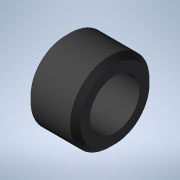
# Autodesk Inventor part: CLBUS5-8-5
Saved by Autodesk Inventor 2021 (Build 250183000, 183)
## iProperties
Created: 2025-06-10
Part Number: CLBUS5-8-5
Material: Generic
Catalog Web Link: www.cadenas.de
Description: CLBU, CLBUB, CLBUM, CLBUS,  CLBP, CLBPB, CLBPM, CLBPS-Bearing Spacers - For Inner Ring
Vendor: MISUMI
Document SubType Name: Modeling
Designer: psAdmin
Manufacturer: MISUMI
Mass: 0.147131 g
Surface Area: 2.50092 cm^2
Volume: 0.147131 cm^3
Density: 1 g/cm^3
Appearance: PSOLRGB-191-191-191
Category: PARTsolutions
Company: MISUMI
Title: CLBUS5-8-5
Author: Cadenas PARTsolutions
Comments: Bearing Spacers - For Inner Ring
PSOL_IDENT_0: {$CADENAS_DATA/23d-libs/misumi/metric/12_bearing_holders/clbu.prj},232 {VTYP=3D},{NB=CLBUS5-8-5},{LI
PSOL_IDENT_1: NA=CLBUS5-8-5},{NN=CLBU, CLBUB, CLBUM, CLBUS,  CLBP, CLBPB, CLBPM, CLBPS},{DATE=09.09.2019 15:26:56}
PSOL_IDENT_2: ,{GEOMDATE=08.10.2015 00:14:34},{VERSION=},{LINEID=30},{WBVAR=LTOL,MAT,ST,DD,L,ALT1},{WBNUMERIC=DD,L
PSOL_IDENT_3: }  {NB=CLBUS5-8-5},{LINA=CLBUS5-8-5},{KT=DUMMY},{PN=CLBUS5-8-5},{TYPE=CLBUS},{TS11=3},{LTOL=M},{MAT=
PSOL_IDENT_4: S},{MATALG= '', 'Aluminum Alloy 5000 series', 'BM', 'Low Carbon Steel', 'S' , 'SUS304' },{ST=},{ST1=
PSOL_IDENT_5: '','-'         },{D=8},{D1=8},{DD=5},{L=5.0},{L1= [1.0:50.0/0.1]},{ALT1=},{ALT1ALG='','w/o LKC (O
PSOL_IDENT_6: verall Length Tolerance)','-LKC','with LKC (Overall Length Tolerance)'},{LTOL1=0/-0.1},{DSS=7},{DD1=
PSOL_IDENT_7: 5},{AP=695ZZ,605ZZ,625ZZ,675ZZ},{LTEMP=.0},{DPN=8},{DSSPN=CLBUS58-5},{ALT1PN=},{DDPN=5},{COLOR=0.75,
PSOL_IDENT_8: 0.75,0.75,0.00}
NB: CLBUS5-8-5
NN: CLBU, CLBUB, CLBUM, CLBUS,  CLBP, CLBPB, CLBPM, CLBPS
NT: Bearing Spacers - For Inner Ring
NBSYN: $PN.
LINA: CLBUS5-8-5
CATALOG: Misumi
PN: CLBUS5-8-5
LTOL: Negative Tolerance
MAT: SUS304
ST: -
D: 8
DD: 5
L: 5
ALT1: w/o LKC (Overall Length Tolerance)
DSS: 7
AP: 695ZZ,605ZZ,625ZZ,675ZZ
SUPPLIER: MISUMI
ARTICLENO: CLBUS5-8-5
BOMINFO: CLBUS5-8-5
CREATOR: CADENAS GmbH
Autodesk Inventor part; units mm, degrees
sketch "Sketch_1" plane through (0, 0, 0) normal (0, 0, 1) x (1, 0, 0)
  line L0 (5, 0) -> (0, 0)
  line L1 (0, 2.5) -> (5, 2.5)
  line L2 (5, 2.5) -> (5, 3.5)
  line L3 (5, 3.5) -> (4.5, 4)
  line L4 (4.5, 4) -> (0.5, 4)
  line L5 (0.5, 4) -> (0, 3.5)
  line L6 (0, 3.5) -> (0, 2.5)
  constraints: 14 end point
revolve "Revolution1" add sketch "Sketch_1" angle 360 about axis through (5, 0, 0) along (1, 0, 0)
ref_plane "to_b_XY" through (0, 0, 0) normal (1, 0, 0) x (0, 0, -1)
ref_plane "to_b_YZ" through (0, 0, 0) normal (0, 0, -1) x (0, 1, 0)
ref_plane "to_b_ZX" through (0, 0, 0) normal (0, 1, 0) x (1, 0, 0)
body "Solid1"
